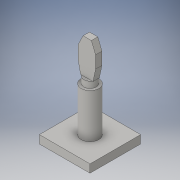
# Autodesk Inventor part: 11mm_Board_Support
Saved by Autodesk Inventor 2016 (Build 200138000, 138)
## iProperties
Created: 2016-09-30
Part Number: 11mm_Board_Support
Material: Generic
Document SubType Name: Modeling
Designer: jfixelle
Density: 1 g/cm^3
Appearance: Default
Author: jfixelle
Autodesk Inventor part; units mm, degrees
ref_plane "YZ Plane" through (0, 0, 0) normal (1, 0, 0) x (0, 1, 0)
ref_plane "XZ Plane" through (0, 0, 0) normal (0, 1, 0) x (-1, 0, 0)
ref_plane "XY Plane" through (0, 0, 0) normal (0, 0, 1) x (1, 0, 0)
sketch "Sketch1" plane through (0, 0, 0) normal (0, 1, 0) x (-1, 0, 0)
  line L0 (6.35, 6.35) -> (-6.35, 6.35)
  line L1 (-6.35, 6.35) -> (-6.35, -6.35)
  line L2 (-6.35, -6.35) -> (6.35, -6.35)
  line L3 (6.35, -6.35) -> (6.35, 6.35)
  point P0 (0, 0)
  dimension "d0" = 12.7
  dimension "d1" = 12.7
  dimension "d2" = 6.35
  dimension "d3" = 6.35
  constraints: 8 end point, 2 parallel, 1 horizontal, 1 perpendicular
  measures "d0" distance of L2.end L0.start
  measures "d1" distance of L1.end L2.end
  measures "d2" distance from line of point (0, 0) L3
  measures "d3" distance from line of point (0, 0) L2
extrude "Extrusion1" add sketch "Sketch1" along normal blind 2.032
sketch "Sketch2" plane through (0, 2.032, 0) normal (0, 1, 0) x (1, 0, 0)
  circle A0 centre (0, 0) radius 2.2
  dimension "d6" = 4.4
  constraints: 1 centre point, 1 coincident
  measures "d6" diameter of A0
extrude "Extrusion2" add sketch "Sketch2" along normal blind 11.1
sketch "Sketch3" plane through (0, 13.132, 0) normal (0, 1, 0) x (1, 0, 0)
  circle A0 centre (0, 0) radius 1.55
  dimension "d9" = 3.1
  constraints: 1 centre point, 1 coincident
  measures "d9" diameter of A0
extrude "Extrusion3" add sketch "Sketch3" along normal blind 1.6
sketch "Sketch4" plane through (0, 0, 0) normal (0, 0, 1) x (1, 0, 0)
  line L0 (-2.2, 23.432) -> (2.2, 23.432)
  line L1 (2.2, 23.432) -> (2.2, 14.732)
  line L2 (2.2, 14.732) -> (-2.2, 14.732)
  line L3 (-2.2, 14.732) -> (-2.2, 23.432)
  line L4 (-6.35, 0) -> (6.35, 0) projected
  line L5 (0, 0) -> (0, -2.1556)
  line L6 (1.55, 14.732) -> (2.2, 17.7603)
  line L7 (1.55, 14.732) -> (-1.55, 14.732) projected
  line L8 (-1.55, 14.732) -> (-2.2, 17.7603)
  line L9 (-0.9244, 23.432) -> (-2.2, 20.8496)
  line L10 (1.1495, 23.432) -> (2.2, 20.8496)
  dimension "d12" = 14.732
  dimension "d13" = 8.7
  dimension "d14" = 4.4
  dimension "d15" = 2.2
  constraints: 18 end point, 7 point on line, 2 parallel, 1 horizontal, 1 perpendicular, 1 vertical
  measures "d12" distance between parallel lines of L4 L2
  measures "d13" distance of L0.end L1.end
  measures "d14" distance between parallel lines of L1 L3
  measures "d15" distance between parallel lines of L1 L5
extrude "Extrusion4" add sketch "Sketch4" along normal mid plane 1.6 contours L0 L10 L1 L6 L2 L8 L3 L9
body "Solid1"
